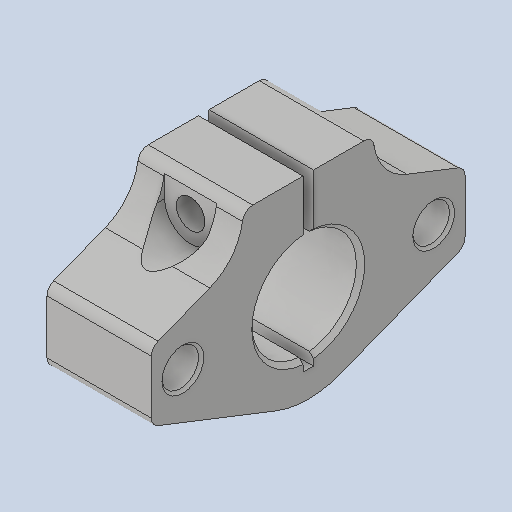
# Autodesk Inventor part: C-SHFMQ20_b
Saved by Autodesk Inventor 2025.2 (Build 292293000, 293)
## iProperties
Category: PARTsolutions
Company: MISUMI
Created: 2023-06-23
Part Number: C-SHFMQ20_b
Material: Generic
Catalog Web Link: www.cadenas.de
Description: C-SHFMQ_base-Economy Shaft Supports - Flanged Slit (Precision Cast) Standard Type
Vendor: MISUMI
Document SubType Name: Modeling
Designer: psAdmin
Manufacturer: MISUMI
Mass: 23.2441 g
Surface Area: 84.2875 cm^2
Volume: 23.2441 cm^3
Density: 1 g/cm^3
Appearance: PSOLRGB-175-175-175
PSOL_IDENT_0: {$CADENAS_DATA/23d-libs/misumi/metric/02_shaft_supports/c_shfmq/c_shfmq_base.prj},166 {VTYP=3D},{NB=
PSOL_IDENT_1: C-SHFMQ20_b},{LINA=C-SHFMQ20},{NN=C-SHFMQ_base},{DATE=12.09.2022 01:30:30},{GEOMDATE=16.03.2021 06:1
PSOL_IDENT_2: 6:05},{VERSION=},{LINEID=40},{WBVAR=},{WBNUMERIC=}  {NB=C-SHFMQ20_b},{LINA=C-SHFMQ20},{KT=DUMMY},{PN=
PSOL_IDENT_3: C-SHFMQ20},{D=20},{L=60},{T=20},{L1=48},{H=37.5},{DD=7.0},{M1=M5},{M=5},{H1=13},{DH=5.5},{R1=17.0},{
PSOL_IDENT_4: R2=10},{R3=2},{L2=25.0},{L3=12.0},{B=2.0},{LH=15.0},{RH=5},{LM=20},{C=0.5}
NB: C-SHFMQ20_b
NN: C-SHFMQ_base
NT: Economy Shaft Supports - Flanged Slit (Precision Cast) Standard Type
NBSYN: $PN._b
LINA: C-SHFMQ20
CATALOG: Misumi
PN: C-SHFMQ20
D: 20
L: 60
T: 20
L1: 48
H: 37.5
DD: 7
M1: M5
SUPPLIER: MISUMI
ARTICLENO: C-SHFMQ20_b
BOMINFO: C-SHFMQ20
CREATOR: CADENAS GmbH
Title: C-SHFMQ20
Author: Cadenas PARTsolutions
Comments: Economy Shaft Supports - Flanged Slit (Precision Cast) Standard Type
Autodesk Inventor part; units mm, degrees
sketch "_____8" plane through (0, 0, 0) normal (1, 0, 0) x (0, 0, -1)
  line L0 (-30, 5.1358) -> (-30, -5.1358)
  arc A0 (-30, -5.1358) -> (-28.7299, -6.9979) centre (-28, -5.1358) ccw
  line L1 (-28.7299, -6.9979) -> (-6.204, -15.8275)
  arc A1 (-6.204, -15.8275) -> (6.204, -15.8275) centre (0, 0) ccw
  line L2 (6.204, -15.8275) -> (28.7299, -6.9979)
  arc A2 (28.7299, -6.9979) -> (30, -5.1358) centre (28, -5.1358) ccw
  line L3 (30, -5.1358) -> (30, 5.1358)
  arc A3 (30, 5.1358) -> (28.7299, 6.9979) centre (28, 5.1358) ccw
  line L4 (28.7299, 6.9979) -> (18.8506, 10.8703)
  arc A4 (12.5986, 18.7801) -> (18.8506, 10.8703) centre (22.5, 20.1806) ccw
  arc A5 (12.5986, 18.7801) -> (10.6183, 20.5) centre (10.6183, 18.5) ccw
  line L5 (10.6183, 20.5) -> (-10.6183, 20.5)
  arc A6 (-10.6183, 20.5) -> (-12.5986, 18.7801) centre (-10.6183, 18.5) ccw
  arc A7 (-18.8506, 10.8703) -> (-12.5986, 18.7801) centre (-22.5, 20.1806) ccw
  line L6 (-18.8506, 10.8703) -> (-28.7299, 6.9979)
  arc A8 (-28.7299, 6.9979) -> (-30, 5.1358) centre (-28, 5.1358) ccw
  constraints: 18 point on circle, 14 end point, 9 centre point
extrude "Extrusion1" add sketch "_____8" along normal blind 20
sketch "_____2" plane through (0, 0, 0) normal (1, 0, 0) x (0, 0, -1)
  line L0 (-1, 37.5) -> (-1, -12)
  line L1 (-1, -12) -> (1, -12)
  line L2 (1, -12) -> (1, 37.5)
  line L3 (1, 37.5) -> (-1, 37.5)
  constraints: 8 end point
extrude "Extrusion2" cut sketch "_____2" along normal blind 20
sketch "_____3" plane through (0, 0, 0) normal (0, 0, 1) x (1, 0, 0)
  line L0 (20, 0) -> (0, 0)
  line L1 (0, 0) -> (0, 10.8)
  line L2 (0, 10.8) -> (0.8, 10)
  line L3 (0.8, 10) -> (19.2, 10)
  line L4 (19.2, 10) -> (20, 10.8)
  line L5 (20, 10.8) -> (20, 0)
  line L6 (20, 0) -> (0, 0)
  constraints: 14 end point
revolve "Revolution1" cut sketch "_____3" angle 360 about axis through (20, 0, 0) along (1, 0, 0)
sketch "_____4" plane through (0, 0, 24) normal (0, 0, 1) x (1, 0, 0)
  line L0 (20, 0) -> (0, 0)
  line L1 (0, 0) -> (0, 4)
  line L2 (0, 4) -> (0.5, 3.5)
  line L3 (0.5, 3.5) -> (19.5, 3.5)
  line L4 (19.5, 3.5) -> (20, 4)
  line L5 (20, 4) -> (20, 0)
  line L6 (20, 0) -> (0, 0)
  constraints: 14 end point
revolve "Revolution2" cut sketch "_____4" angle 360 about axis through (20, 0, 24) along (1, 0, 0)
pattern_linear "Rectangular Pattern1" count 2 spacing 48 along (0, 0, -1) of "Revolution2"
sketch "Sketch5" plane through (0, 20.5, -1) normal (0, 0, 1) x (1, 0, 0)
  point P0 (10, -5.5)
hole "Hole1" at (10, 15, -1) direction (0, 0, -1) diameter 4.134 depth 16.5 countersink diameter 5 countersink angle 90 thread size "M5x0.8" class "6H" standard "ISO Metric profile"
sketch "Sketch6" plane through (20, 20.5, 1) normal (0, 0, -1) x (-1, 0, 0)
  point P0 (10, -5.5)
hole "Hole2" at (10, 15, 1) direction (0, 0, 1) diameter 5.5 depth 25
sketch "_____9" plane through (0, 0, 12.5) normal (0, 0, 1) x (1, 0, 0)
  line L0 (5, 33.75) -> (5, 15)
  arc A0 (5, 15) -> (15, 15) centre (10, 15) ccw
  line L1 (15, 15) -> (15, 33.75)
  line L2 (15, 33.75) -> (5, 33.75)
  constraints: 6 end point, 2 point on circle, 1 centre point
extrude "Extrusion3" cut sketch "_____9" along normal blind 20
ref_plane "to_bolt_XY" through (10, 15, 12.5) normal (0, 0, 1) x (1, 0, 0)
ref_plane "to_bolt_YZ" through (10, 15, 12.5) normal (1, 0, 0) x (0, 1, 0)
ref_plane "to_bolt_ZX" through (10, 15, 12.5) normal (0, 1, 0) x (0, 0, 1)
body "Solid1"
